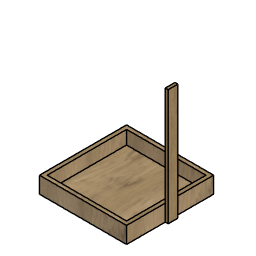
Hammer Head Base (Autodesk Fusion 360 design; units mm, degrees)
Autodesk Fusion 360 part; units mm, degrees
sketch "草图1" plane through (0, 0, 0) normal (0, 0, 1) x (1, 0, 0) in component "base"
  line L0 (200, -200) -> (-200, -200) construction
  line L1 (-200, -200) -> (-200, 200) construction
  line L2 (-200, 200) -> (200, 200) construction
  line L3 (200, 200) -> (200, -200) construction
  line L4 (200, -200) -> (-200, 200) construction
  line L5 (-200, -200) -> (200, 200) construction
  line L6 (205, -205) -> (-205, -205)
  line L7 (-205, -205) -> (-205, 205)
  line L8 (-205, 205) -> (205, 205)
  line L9 (205, 205) -> (205, -205)
  line L10 (225, -225) -> (-225, -225)
  line L11 (-225, -225) -> (-225, 225)
  line L12 (-225, 225) -> (225, 225)
  line L13 (225, 225) -> (225, -225)
  line L14 (225, -25) -> (240, -25)
  line L15 (240, -25) -> (240, 25)
  line L16 (240, 25) -> (225, 25)
  line L17 (225, 25) -> (225, -25)
  line L18 (1.75, 0) -> (22.5, 0)
  dimension "d1" = 400
  dimension "d2" = 400
  dimension "d3" = -5
  dimension "d4" = -25
  dimension "d9" = 15
  dimension "d10" = 50
  constraint horizontal L0
  constraint perpendicular L0 L1
  constraint parallel L0 L2
  constraint parallel L1 L3
  constraint coincident L4 origin
  constraint coincident L5 origin
  constraint horizontal L14
  constraint vertical L15
  constraint horizontal L16
  constraint vertical L17
  constraint coincident L13 L14.start
  constraint symmetric L14 L16 L18
  measures "d1" distance of L1.end L2.end
  measures "d2" distance of L0.end L1.end
  measures "d9" distance of L14.start L14.end
  measures "d10" distance of L14.start L16.end
extrude "拉伸1" add sketch "草图1" along normal blind 85 contours L10 L11 L12 L13 L17 makes body 1 in component "base"
extrude "拉伸2" add sketch "草图1" along normal blind 15 contours L6 L7 L8 L9 bodies 1 in component "base"
extrude "拉伸3" add sketch "草图1" along normal blind 600 separate body contours L13 L14 L15 L16 L17 makes body 2 in component "base"
component "base" placed x (1, 0, 0) y (0, 1, 0) z (0, 0, 1) at (0, 0, 0)
